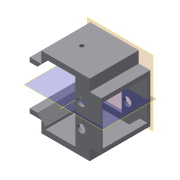
# Autodesk Inventor part: 30_Cube_Z_Focus_Drylin_manual_base_v3
Saved by Autodesk Inventor 2019.4 (Build 234330000, 330)
## iProperties
Created: 2021-04-25
Part Number: 30_Cube_Z_Focus_Drylin_manual_base_v3
Material: Generic
Document SubType Name: Modeling
Designer: diederichbenedict
Density: 1 g/cm^3
Appearance: Default
Author: diederichbenedict
Autodesk Inventor part; units mm, degrees
ref_plane "Work Plane1" through (0, 0, 0) normal (0, 0, 1) x (1, 0, 0)
sketch "Sketch1" plane through (0, 0, 0) normal (0, 0, 1) x (1, 0, 0)
  arc A0 (12.5934, -5.8404) -> (12.8401, -5.9947) centre (12.8241, -5.7459) ccw construction
  line L0 (12.8401, -5.9947) -> (16.4715, -5.9947) construction
  line L1 (16.4715, -5.9947) -> (16.97, -5.4961) construction
  line L2 (16.97, -5.4961) -> (16.97, 1.583) construction
  arc A1 (16.97, 2.3806) -> (16.97, 1.583) centre (17.2691, 1.9818) ccw construction
  line L3 (16.97, 2.3806) -> (16.97, 5.4715) construction
  line L4 (16.97, 5.4715) -> (16.4715, 5.97) construction
  line L5 (16.4715, 5.97) -> (12.8401, 5.97) construction
  arc A2 (12.8401, 5.97) -> (12.6094, 5.8152) centre (12.8401, 5.7207) ccw construction
  arc A3 (12.0954, 5.2394) -> (12.6094, 5.8152) centre (11.5075, 6.2814) ccw construction
  arc A4 (12.0954, 5.2394) -> (11.974, 5.0466) centre (12.2223, 5.0248) ccw construction
  line L6 (11.974, 5.0466) -> (11.9439, 4.702) construction
  arc A5 (11.6955, 4.4744) -> (11.9439, 4.702) centre (11.6955, 4.7237) ccw construction
  line L7 (11.6955, 4.4744) -> (11.2445, 4.4744) construction
  arc A6 (10.9961, 4.702) -> (11.2445, 4.4744) centre (11.2445, 4.7237) ccw construction
  line L8 (10.9961, 4.702) -> (10.9642, 5.0674) construction
  arc A7 (10.9642, 5.0674) -> (10.8487, 5.2566) centre (10.7158, 5.0457) ccw construction
  arc A8 (10.3792, 5.8152) -> (10.8487, 5.2566) centre (11.4862, 6.2691) ccw construction
  arc A9 (10.3792, 5.8152) -> (10.1485, 5.97) centre (10.1485, 5.7206) ccw construction
  line L9 (10.1485, 5.97) -> (9.4685, 5.97) construction
  line L10 (9.4685, 5.97) -> (8.97, 5.4715) construction
  line L11 (8.97, 5.4715) -> (8.97, -5.4961) construction
  line L12 (8.97, -5.4961) -> (9.4685, -5.9947) construction
  line L13 (9.4685, -5.9947) -> (10.1412, -5.9947) construction
  arc A10 (10.1412, -5.9947) -> (10.3791, -5.84) centre (10.1485, -5.7455) ccw construction
  arc A11 (10.8487, -5.2813) -> (10.3791, -5.84) centre (11.4862, -6.2938) ccw construction
  arc A12 (10.8487, -5.2813) -> (10.9642, -5.0921) centre (10.7158, -5.0704) ccw construction
  line L14 (10.9642, -5.0921) -> (10.9961, -4.7266) construction
  arc A13 (11.2445, -4.4991) -> (10.9961, -4.7266) centre (11.2445, -4.7483) ccw construction
  line L15 (11.2445, -4.4991) -> (11.6955, -4.4991) construction
  arc A14 (11.9439, -4.7266) -> (11.6955, -4.4991) centre (11.6955, -4.7483) ccw construction
  line L16 (11.9439, -4.7266) -> (11.974, -5.0712) construction
  arc A15 (11.974, -5.0712) -> (12.0954, -5.264) centre (12.2223, -5.0495) ccw construction
  arc A16 (12.5934, -5.8404) -> (12.0954, -5.264) centre (11.4862, -6.2938) ccw construction
  arc A17 (24.85, 22.85) -> (22.85, 24.85) centre (22.85, 22.85) ccw construction
  line L17 (22.85, 24.85) -> (-16.97, 24.85) construction
  line L18 (-16.97, 24.85) -> (-16.97, 21.15) construction
  line L19 (-16.97, 21.15) -> (16.97, 21.15) construction
  line L20 (16.97, 16.97) -> (16.97, 21.15) construction
  line L21 (21.15, 16.97) -> (16.97, 16.97) construction
  line L22 (21.15, 16.97) -> (21.15, -16.97) construction
  line L23 (21.15, -16.97) -> (24.85, -16.97) construction
  line L24 (24.85, -16.97) -> (24.85, 22.85) construction
  line L25 (23.75, 23.25) -> (23.75, 18.15) construction
  arc A18 (23.25, 17.65) -> (23.75, 18.15) centre (23.25, 18.15) ccw construction
  line L26 (23.25, 17.65) -> (20.8937, 17.65) construction
  arc A19 (20.5239, 17.8134) -> (20.8937, 17.65) centre (20.8937, 18.15) ccw construction
  line L27 (20.5239, 17.8134) -> (17.7803, 20.8273) construction
  arc A20 (17.65, 21.1639) -> (17.7803, 20.8273) centre (18.15, 21.1639) ccw construction
  line L28 (17.65, 21.1639) -> (17.65, 23.25) construction
  arc A21 (18.15, 23.75) -> (17.65, 23.25) centre (18.15, 23.25) ccw construction
  line L29 (18.15, 23.75) -> (23.25, 23.75) construction
  arc A22 (23.75, 23.25) -> (23.25, 23.75) centre (23.25, 23.25) ccw construction
  arc A23 (-24.85, -22.85) -> (-22.85, -24.85) centre (-22.85, -22.85) ccw construction
  line L30 (-22.85, -24.85) -> (16.97, -24.85) construction
  line L31 (16.97, -24.85) -> (16.97, -21.15) construction
  line L32 (16.97, -21.15) -> (-16.97, -21.15) construction
  line L33 (-16.97, -16.97) -> (-16.97, -21.15) construction
  line L34 (-21.15, -16.97) -> (-16.97, -16.97) construction
  line L35 (-21.15, -16.97) -> (-21.15, 16.97) construction
  line L36 (-21.15, 16.97) -> (-24.85, 16.97) construction
  line L37 (-24.85, 16.97) -> (-24.85, -22.85) construction
  line L38 (-20.8273, -17.7803) -> (-17.8134, -20.5239) construction
  arc A24 (-17.65, -20.8937) -> (-17.8134, -20.5239) centre (-18.15, -20.8937) ccw construction
  line L39 (-17.65, -20.8937) -> (-17.65, -23.25) construction
  arc A25 (-18.15, -23.75) -> (-17.65, -23.25) centre (-18.15, -23.25) ccw construction
  line L40 (-18.15, -23.75) -> (-23.25, -23.75) construction
  arc A26 (-23.75, -23.25) -> (-23.25, -23.75) centre (-23.25, -23.25) ccw construction
  line L41 (-23.75, -23.25) -> (-23.75, -18.15) construction
  arc A27 (-23.25, -17.65) -> (-23.75, -18.15) centre (-23.25, -18.15) ccw construction
  line L42 (-23.25, -17.65) -> (-21.1639, -17.65) construction
  arc A28 (-20.8273, -17.7803) -> (-21.1639, -17.65) centre (-21.1639, -18.15) ccw construction
  arc A29 (-22.85, 24.85) -> (-24.85, 22.85) centre (-22.85, 22.85) ccw construction
  line L43 (-22.85, 24.85) -> (16.97, 24.85) construction
  line L44 (16.97, 24.85) -> (16.97, 21.15) construction
  line L45 (16.97, 21.15) -> (-16.97, 21.15) construction
  line L46 (-16.97, 16.97) -> (-16.97, 21.15) construction
  line L47 (-21.15, 16.97) -> (-16.97, 16.97) construction
  line L48 (-21.15, 16.97) -> (-21.15, -16.97) construction
  line L49 (-21.15, -16.97) -> (-24.85, -16.97) construction
  line L50 (-24.85, -16.97) -> (-24.85, 22.85) construction
  line L51 (-20.8273, 17.7803) -> (-17.8134, 20.5239) construction
  arc A30 (-17.8134, 20.5239) -> (-17.65, 20.8937) centre (-18.15, 20.8937) ccw construction
  line L52 (-17.65, 20.8937) -> (-17.65, 23.25) construction
  arc A31 (-17.65, 23.25) -> (-18.15, 23.75) centre (-18.15, 23.25) ccw construction
  line L53 (-18.15, 23.75) -> (-23.25, 23.75) construction
  arc A32 (-23.25, 23.75) -> (-23.75, 23.25) centre (-23.25, 23.25) ccw construction
  line L54 (-23.75, 23.25) -> (-23.75, 18.15) construction
  arc A33 (-23.75, 18.15) -> (-23.25, 17.65) centre (-23.25, 18.15) ccw construction
  line L55 (-23.25, 17.65) -> (-21.1639, 17.65) construction
  arc A34 (-21.1639, 17.65) -> (-20.8273, 17.7803) centre (-21.1639, 18.15) ccw construction
  arc A35 (22.85, -24.85) -> (24.85, -22.85) centre (22.85, -22.85) ccw construction
  line L56 (22.85, -24.85) -> (-16.97, -24.85) construction
  line L57 (-16.97, -24.85) -> (-16.97, -21.15) construction
  line L58 (-16.97, -21.15) -> (16.97, -21.15) construction
  line L59 (16.97, -16.97) -> (16.97, -21.15) construction
  line L60 (21.15, -16.97) -> (16.97, -16.97) construction
  line L61 (21.15, -16.97) -> (21.15, 16.97) construction
  line L62 (21.15, 16.97) -> (24.85, 16.97) construction
  line L63 (24.85, 16.97) -> (24.85, -22.85) construction
  line L64 (23.75, -23.25) -> (23.75, -18.15) construction
  arc A36 (23.75, -18.15) -> (23.25, -17.65) centre (23.25, -18.15) ccw construction
  line L65 (23.25, -17.65) -> (20.8937, -17.65) construction
  arc A37 (20.8937, -17.65) -> (20.5239, -17.8134) centre (20.8937, -18.15) ccw construction
  line L66 (20.5239, -17.8134) -> (17.7803, -20.8273) construction
  arc A38 (17.7803, -20.8273) -> (17.65, -21.1639) centre (18.15, -21.1639) ccw construction
  line L67 (17.65, -21.1639) -> (17.65, -23.25) construction
  arc A39 (17.65, -23.25) -> (18.15, -23.75) centre (18.15, -23.25) ccw construction
  line L68 (18.15, -23.75) -> (23.25, -23.75) construction
  arc A40 (23.25, -23.75) -> (23.75, -23.25) centre (23.25, -23.25) ccw construction
  circle A41 centre (0.47, -10.47) radius 1.1 construction
  circle A42 centre (0.47, 12.53) radius 1.025 construction
  line L69 (24.85, 16.87) -> (16.87, 16.87)
  line L70 (16.87, 16.87) -> (16.87, -16.87)
  line L71 (16.87, -16.87) -> (24.85, -16.87)
  line L72 (24.85, -16.87) -> (24.85, 16.87)
  line L73 (-16.87, 24.85) -> (16.87, 24.85)
  line L74 (16.87, 24.85) -> (16.87, 16.87)
  line L75 (16.87, 16.87) -> (-16.87, 16.87)
  line L76 (-16.87, 16.87) -> (-16.87, 24.85)
  line L77 (-16.87, 16.87) -> (-24.85, 16.87)
  line L78 (-24.85, 16.87) -> (-24.85, -16.87)
  line L79 (-24.85, -16.87) -> (-16.87, -16.87)
  line L80 (-16.87, -16.87) -> (-16.87, 16.87)
  line L81 (-16.87, -24.85) -> (16.87, -24.85)
  line L82 (16.87, -24.85) -> (16.87, -16.87)
  line L83 (16.87, -16.87) -> (-16.87, -16.87)
  line L84 (-16.87, -16.87) -> (-16.87, -24.85)
  circle A43 centre (10.75, 8) radius 3 projected
  circle A44 centre (10.75, -8) radius 3 projected
  line L85 (16.87, 16.87) -> (6.87, 16.87)
  line L86 (6.87, 16.87) -> (6.87, -16.87)
  line L87 (6.87, -16.87) -> (16.87, -16.87)
  line L88 (16.87, -16.87) -> (16.87, 16.87)
  point P0 (0, 0)
  dimension "d1" = 0.1
  dimension "d2" = 0.1
  dimension "d3" = 0.1
  dimension "d4" = 0.1
  dimension "d5" = 0.1
  dimension "d6" = 0
  dimension "d7" = 0
  dimension "d90" = 10
  dimension "d91" = 33.74
  constraints: 40 end point, 10 parallel, 10 point on line, 5 horizontal, 5 perpendicular
  measures "d1" distance between parallel lines of L47 L77
  measures "d2" distance between parallel lines of L18 L76
  measures "d3" distance between parallel lines of L44 L74
  measures "d4" distance between parallel lines of L60 L71
  measures "d5" distance between parallel lines of L33 L84
  measures "d6" distance between parallel lines of L77 L75
  measures "d7" distance between parallel lines of L79 L83
  measures "d90" distance of L87.end L86.end
  measures "d91" distance of L86.end L85.end
extrude "Extrusion1" add sketch "Sketch1" along normal blind 2 contours L72 L71 L70 L69 | L75 L76 L73 L74 | L70 L83 L86 L75 | L82 L81 L84 L83 | L80 L79 L78 L77
chamfer "Chamfer1" [suppressed]
sketch "Sketch2" plane through (0, 0, 2) normal (0, 0, 1) x (1, 0, 0)
  line L0 (-16.87, -16.87) -> (-16.87, 16.87) projected
  line L1 (-16.87, 16.87) -> (6.87, 16.87) projected
  line L2 (6.87, -16.87) -> (-16.87, -16.87) projected
  line L3 (-16.87, -16.87) -> (-16.87, -24.85) projected
  line L4 (-16.87, -24.85) -> (16.87, -24.85) projected
  line L5 (16.87, -24.85) -> (16.87, -16.87) projected
  line L6 (16.87, -16.87) -> (24.85, -16.87) projected
  line L7 (24.85, -16.87) -> (24.85, 16.87) projected
  line L8 (24.85, 16.87) -> (16.87, 16.87) projected
  line L9 (16.87, 16.87) -> (16.87, 24.85) projected
  line L10 (16.87, 24.85) -> (-16.87, 24.85) projected
  line L11 (-16.87, 24.85) -> (-16.87, 16.87) projected
  line L12 (-16.87, 16.87) -> (-24.85, 16.87) projected
  line L13 (-24.85, 16.87) -> (-24.85, -16.87) projected
  line L14 (-24.85, -16.87) -> (-16.87, -16.87) projected
  line L15 (13.8689, -19.5269) -> (13.8689, -21.8489)
  line L16 (-13.8689, -21.8489) -> (-13.8689, -19.5269)
  line L17 (-13.8689, -19.5269) -> (-19.5269, -13.8689)
  line L18 (-19.5269, -13.8689) -> (-21.8489, -13.8689)
  line L19 (-21.8489, 13.8689) -> (-19.5269, 13.8689)
  line L20 (-19.5269, 13.8689) -> (-13.8689, 19.5269)
  line L21 (-13.8689, 19.5269) -> (-13.8689, 21.8489)
  line L22 (13.8689, 21.8489) -> (13.8689, 19.5269)
  line L23 (13.8689, 19.5269) -> (19.5269, 13.8689)
  line L24 (19.5269, 13.8689) -> (21.8489, 13.8689)
  line L25 (21.8489, -13.8689) -> (19.5269, -13.8689)
  line L26 (19.5269, -13.8689) -> (13.8689, -19.5269)
  line L27 (13.8689, -21.8489) -> (13.8689, -24.85)
  line L28 (16.87, -24.85) -> (-16.87, -24.85) projected
  line L29 (21.8489, -13.8689) -> (24.85, -13.8689)
  line L30 (24.85, -16.87) -> (24.85, 16.87) projected
  line L31 (21.8489, 13.8689) -> (24.85, 13.8689)
  line L32 (13.8689, 21.8489) -> (13.8689, 24.85)
  line L33 (-13.8689, 21.8489) -> (-13.8689, 24.85)
  line L34 (-21.8489, 13.8689) -> (-24.85, 13.8689)
  line L35 (-21.8489, -13.8689) -> (-24.85, -13.8689)
  line L36 (-13.8689, -21.8489) -> (-13.8689, -24.85)
  line L37 (13.8689, -21.8489) -> (11.5469, -21.8489)
  line L38 (-11.5469, -21.8489) -> (-13.8689, -21.8489)
  line L39 (21.8489, 13.8689) -> (21.8489, 11.5469)
  line L40 (21.8489, -11.5469) -> (21.8489, -13.8689)
  line L41 (-21.8489, -13.8689) -> (-21.8489, -11.5469)
  line L42 (-21.8489, 11.5469) -> (-21.8489, 13.8689)
  line L43 (-13.8689, 21.8489) -> (-11.5469, 21.8489)
  line L44 (11.5469, 21.8489) -> (13.8689, 21.8489)
  line L45 (6.87, 16.87) -> (6.87, -16.87) projected
  point P0 (0, 0)
  dimension "d13" = 3.0011
  constraints: 56 end point, 20 point on line, 3 perpendicular, 1 parallel
  measures "d13" distance between parallel lines of L5 L15
ref_plane "Work Plane2" through (-16.97, -24.85, 34.1) normal (0, 0, -1) x (0, 1, 0)
extrude "Extrusion2" add sketch "Sketch2" along normal up to surface (32.1 mm away) contours L27 L15 L26 L25 L29 L7 L6 L5 L4
pattern_circular "Circular Pattern1" count 4 over 360 about axis through (0, 0, 17.13) along (0, 0, -1) of "Extrusion2"
sketch "Sketch3" plane through (-24.85, -13.8689, 34.1) normal (0, 0, 1) x (1, 0, 0)
  circle A0 centre (13.82, 14.8989) radius 1.5 projected
  line L0 (10.9811, -5.658) -> (5.3231, 0) projected
  line L1 (5.3231, 0) -> (0, 0) projected
  line L2 (0, 0) -> (0, -3.0011) projected
  line L3 (0, -3.0011) -> (7.98, -3.0011) projected
  line L4 (7.98, -3.0011) -> (7.98, -10.9811) projected
  line L5 (7.98, -10.9811) -> (10.9811, -10.9811) projected
  line L6 (10.9811, -10.9811) -> (10.9811, -5.658) projected
  line L7 (5.3231, 27.7378) -> (10.9811, 33.3958) projected
  line L8 (10.9811, 33.3958) -> (10.9811, 38.7189) projected
  line L9 (10.9811, 38.7189) -> (7.98, 38.7189) projected
  line L10 (7.98, 38.7189) -> (7.98, 30.7389) projected
  line L11 (7.98, 30.7389) -> (0, 30.7389) projected
  line L12 (0, 30.7389) -> (0, 27.7378) projected
  line L13 (0, 27.7378) -> (5.3231, 27.7378) projected
  line L14 (10.9811, -10.9811) -> (16.9811, -10.9811)
  line L15 (16.9811, 38.7189) -> (10.9811, 38.7189)
  line L16 (0, 0) -> (0, 27.7378)
  line L17 (0, 0) -> (5.3231, 0)
  line L18 (5.3231, 0) -> (5.3231, 27.7378)
  line L19 (5.3231, 27.7378) -> (0, 27.7378)
  line L20 (0, 27.7378) -> (0, 0)
  line L21 (5.3231, 0) -> (0, 0) projected
  line L22 (5.3231, 0) -> (10.9811, -5.658)
  line L23 (10.9811, 33.3958) -> (5.3231, 27.7378)
  line L24 (38.7189, 38.7189) -> (38.7189, 33.3958) projected
  line L25 (38.7189, -5.658) -> (38.7189, -10.9811) projected
  line L26 (10.9811, -10.9811) -> (38.7189, -10.9811)
  line L27 (38.7189, -10.9811) -> (38.7189, -5.658)
  line L28 (38.7189, -5.658) -> (10.9811, -5.658)
  line L29 (10.9811, -5.658) -> (10.9811, -10.9811)
  line L30 (10.9811, 38.7189) -> (10.9811, 33.3958) projected
  line L31 (10.9811, 38.7189) -> (38.7189, 38.7189)
  line L32 (38.7189, 38.7189) -> (38.7189, 33.3958)
  line L33 (38.7189, 33.3958) -> (10.9811, 33.3958)
  line L34 (10.9811, 33.3958) -> (10.9811, 38.7189)
  line L35 (16.9811, -10.9811) -> (16.9811, -5.658)
  line L36 (16.9811, 33.3958) -> (16.9811, 38.7189)
  line L37 (10.9811, 38.7189) -> (10.9811, 33.3958)
  line L38 (10.9811, -5.658) -> (10.9811, -10.9811)
  line L39 (10.9811, -5.658) -> (10.9811, 0)
  line L40 (10.9811, 27.7378) -> (10.9811, 33.3958)
  line L41 (49.7, 0) -> (44.3769, 0) projected
  line L42 (44.3769, 27.7378) -> (49.7, 27.7378) projected
  line L43 (44.3769, 27.7378) -> (49.7, 27.7378)
  line L44 (49.7, 27.7378) -> (49.7, 0)
  line L45 (49.7, 0) -> (44.3769, 0)
  line L46 (44.3769, 0) -> (44.3769, 27.7378)
  point P0 (24.85, 13.8689)
  dimension "d19" = 6
  constraints: 54 end point, 14 equal length, 6 perpendicular, 5 horizontal, 4 point on line, 3 vertical
  measures "d19" distance of L15.end L15.start
extrude "Extrusion3" add sketch "Sketch3" against normal blind 1 contours L6 L5 L4 L3 L2 L1 L0 | L13 L12 L11 L10 L9 L8 L7 | L41 L46 L42 L44
ref_plane "Work Plane3" through (16.97, -5.4961, -37.9) normal (1, 0, 0) x (0, 1, 0)
ref_plane "Work Plane4" through (-25.03, -12.97, -12) normal (0, 0, 1) x (1, 0, 0)
sketch "Sketch14" plane through (-16.87, 24.85, 0) normal (0, 1, 0) x (1, 0, 0)
  line L0 (3.0011, -2) -> (3.0011, -34.1) projected
  line L1 (30.7389, -2) -> (3.0011, -2) projected
  line L2 (30.7389, -2) -> (30.7389, -34.1) projected
  line L3 (33.74, 0) -> (33.74, -34.1) projected
  line L4 (33.74, 0) -> (0, 0) projected
  line L5 (0, 0) -> (0, -34.1) projected
  line L6 (3.0011, -34.1) -> (0, -34.1) projected
  line L7 (3.0011, -2) -> (3.0011, -34.1) projected
  line L8 (30.7389, -34.1) -> (36.3969, -34.1) projected
  line L9 (3.0011, -2) -> (30.7389, -2)
  line L10 (30.7389, -2) -> (30.7389, -34.1)
  line L11 (30.7389, -34.1) -> (3.0011, -34.1)
  line L12 (3.0011, -34.1) -> (3.0011, -2)
  circle A0 centre (11.8112, -17.0464) radius 1.4 construction
  circle A1 centre (11.2546, -17.0464) radius 1.4
  line L13 (33.74, -34.1) -> (30.7389, -34.1) projected
  point P0 (16.87, 0)
  dimension "d89" = 2.8
  constraints: 8 end point, 2 parallel, 1 centre point, 1 horizontal, 1 perpendicular
  measures "d89" diameter of A1
extrude "Extrusion12" add sketch "Sketch14" against normal up to surface (3.7 mm away) contours L1 L2 L11 L0
ref_plane "Work Plane5" through (-24.85, 0, 0) normal (0, -1, 0) x (1, 0, 0)
mirror "Mirror1" about plane through (-24.85, 0, 0) normal (0, -1, 0) of "Extrusion12"
sketch "Sketch16" plane through (-16.87, -24.85, 34.1) normal (0, 0, 1) x (1, 0, 0)
  line L0 (0, 0) -> (33.74, 0) projected
  line L1 (33.74, 0) -> (33.74, 7.98) projected
  line L2 (33.74, 7.98) -> (41.72, 7.98) projected
  line L3 (41.72, 7.98) -> (41.72, 41.72) projected
  line L4 (3.0011, 44.3769) -> (3.0011, 46) projected
  line L5 (30.7389, 46) -> (3.0011, 46) projected
  line L6 (30.7389, 46) -> (30.7389, 44.3769) projected
  line L7 (30.7389, 44.3769) -> (36.3969, 38.7189) projected
  line L8 (36.3969, 38.7189) -> (36.3969, 10.9811) projected
  line L9 (36.3969, 10.9811) -> (30.7389, 5.3231) projected
  line L10 (30.7389, 5.3231) -> (30.7389, 3.7) projected
  line L11 (30.7389, 3.7) -> (3.0011, 3.7) projected
  line L12 (3.0011, 3.7) -> (3.0011, 5.3231) projected
  circle A0 centre (27.62, 16.85) radius 3 projected
  circle A1 centre (27.62, 32.85) radius 3 projected
  line L13 (0, 7.98) -> (-7.98, 7.98) projected
  line L14 (-7.98, 7.98) -> (-7.98, 41.72) projected
  line L15 (-7.98, 41.72) -> (0, 41.72) projected
  line L16 (0, 49.7) -> (0, 41.72) projected
  line L17 (33.74, 49.7) -> (0, 49.7) projected
  line L18 (33.74, 41.72) -> (33.74, 49.7) projected
  line L19 (41.72, 41.72) -> (33.74, 41.72) projected
  line L20 (41.72, 7.98) -> (41.72, 41.72) projected
  line L21 (41.72, 7.98) -> (33.74, 7.98) projected
  line L22 (33.74, 7.98) -> (33.74, 0) projected
  line L23 (33.74, 0) -> (0, 0) projected
  line L24 (0, 0) -> (0, 7.98) projected
  line L25 (0, 7.98) -> (23.74, 7.98) projected
  line L26 (23.74, 7.98) -> (23.74, 41.72) projected
  line L27 (0, 41.72) -> (23.74, 41.72) projected
  line L28 (0, 41.72) -> (0, 7.98) projected
  line L29 (23.74, 41.72) -> (23.74, 46)
  line L30 (30.7389, 46) -> (3.0011, 46) projected
  line L31 (23.74, 7.98) -> (23.74, 3.7)
  line L32 (30.7389, 3.7) -> (3.0011, 3.7) projected
  line L33 (-2.6569, 10.9811) -> (-7.98, 10.9811) projected
  line L34 (-7.98, 10.9811) -> (-7.98, 7.98) projected
  line L35 (-7.98, 7.98) -> (0, 7.98) projected
  line L36 (0, 7.98) -> (0, 0) projected
  line L37 (41.72, 41.72) -> (33.74, 41.72) projected
  line L38 (33.74, 41.72) -> (33.74, 49.7) projected
  line L39 (33.74, 49.7) -> (0, 49.7) projected
  line L40 (0, 49.7) -> (0, 41.72) projected
  line L41 (0, 41.72) -> (-7.98, 41.72) projected
  line L42 (-7.98, 41.72) -> (-7.98, 38.7189) projected
  line L43 (-7.98, 38.7189) -> (-2.6569, 38.7189) projected
  line L44 (-2.6569, 38.7189) -> (3.0011, 44.3769) projected
  line L45 (3.0011, 5.3231) -> (-2.6569, 10.9811) projected
  point P0 (16.87, 24.85)
  constraints: 4 end point, 3 point on line, 1 perpendicular
extrude "Extrusion14" add sketch "Sketch16" against normal blind 2 contours L26 L29 L5 L6 L7 L8 L9 L10 L11 L31
equation "\"d2\" = d1"
equation "\"d3\" = d1"
equation "\"d4\" = d1"
equation "\"d5\" = d1"
body "Solid1"
